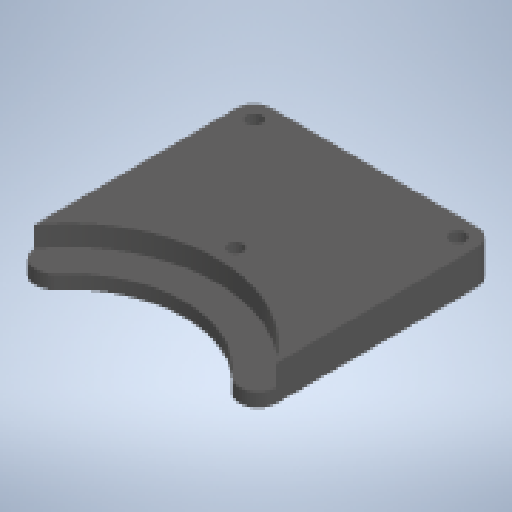
# Autodesk Inventor part: waist_cover
Saved by Autodesk Inventor 2024.1 (Build 281209000, 209)
## iProperties
Created: 2024-02-14
Part Number: waist_cover
Material: 一般
Document SubType Name: Modeling
Designer: hibik
Density: 1 g/cm^3
Appearance: 既定
Author: hibik
Autodesk Inventor part; units mm, degrees
ref_plane "YZ Plane" through (0, 0, 0) normal (1, 0, 0) x (0, 1, 0)
ref_plane "XZ Plane" through (0, 0, 0) normal (0, 1, 0) x (-1, 0, 0)
ref_plane "XY Plane" through (0, 0, 0) normal (0, 0, 1) x (1, 0, 0)
sketch "スケッチ1" plane through (0, 0, 0) normal (0, 1, 0) x (-1, 0, 0)
  circle A0 centre (0, 0) radius 12.5
  line L0 (13, 0) -> (-13, 0)
  line L1 (-13, 0) -> (-13, -33)
  line L2 (-13, -33) -> (13, -33)
  line L3 (13, -33) -> (13, 0)
  circle A1 centre (0, 0) radius 16
  circle A2 centre (11, -31) radius 0.8
  circle A3 centre (-11, -31) radius 0.8
  circle A4 centre (0, -18) radius 0.8
  line L4 (0, -42.8) -> (0, 25.8) projected
  point P0 (13, -9.3274)
  point P1 (-13, -9.3274)
  point P2 (12.5, 0)
  point P3 (-12.5, 0)
  dimension "d0" = 25
  dimension "d1" = 26
  dimension "d2" = 33
  dimension "d3" = 32
  dimension "d9" = 1.6
  dimension "d10" = 1.6
  dimension "d11" = 2
  dimension "d12" = 2
  dimension "d13" = 2
  dimension "d14" = 2
  dimension "d15" = 1.6
  dimension "d16" = 15
  constraints: 8 end point, 5 centre point, 5 coincident, 2 parallel, 1 horizontal, 1 midpoint, 1 perpendicular, 1 point on line
  measures "d0" diameter of A0
  measures "d1" distance of L0.start L0.end
  measures "d2" distance of L2.end L0.start
  measures "d3" diameter of A1
  measures "d9" diameter of A2
  measures "d10" diameter of A3
  measures "d11" distance from line of L3 A2.centre
  measures "d12" distance from line of L2 A2.centre
  measures "d13" distance from line of L2 A3.centre
  measures "d14" distance from line of L1 A3.centre
  measures "d15" diameter of A4
  measures "d16" distance from line of L2 A4.centre
extrude "押し出し1" add sketch "スケッチ1" along normal blind 3.75 contours L4 A4 L2 L1 A1 | A1 L3 L2 L4 A4
extrude "押し出し2" add sketch "スケッチ1" along normal blind 1.5 contours L0 L3 A1 L4 A0 | L4 A1 L1 L0 A0 picked at (2.1799, -14.5796) picked at (-2.1799, -14.5796)
fillet "フィレット1" radius 2 6 edges at (-13, 0.75, 0) (-12.5, 0.75, 0) (13, 0.75, 0) (12.5, 0.75, 0) (13, 1.875, -33) (-13, 1.875, -33)
